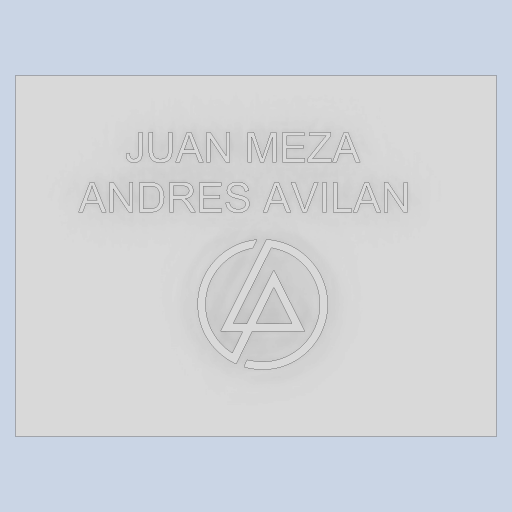
# Autodesk Inventor part: WorkObject
Saved by Autodesk Inventor 2024 (Build 280153000, 153)
## iProperties
Created: 2025-06-12
Part Number: WorkObject
Material: Genérico
Document SubType Name: Modeling
Designer: ANDRES
Density: 1 g/cm^3
Appearance: Valor por defecto
Author: ANDRES
## iProperties of the stored document WorkObject_3DPrint.ipt
Created: 2025-06-12
Part Number: WorkObject_3DPrint
Material: Genérico
Document SubType Name: Modeling
Designer: ANDRES
Density: 1 g/cm^3
Appearance: Valor por defecto
Author: ANDRES
Autodesk Inventor part; units mm, degrees
(part 1 of 2)
ref_plane "YZ Plane" through (0, 0, 0) normal (1, 0, 0) x (0, 1, 0)
ref_plane "XZ Plane" through (0, 0, 0) normal (0, 1, 0) x (-1, 0, 0)
ref_plane "XY Plane" through (0, 0, 0) normal (0, 0, 1) x (1, 0, 0)
sketch "Boceto1" plane through (0, 0, 0) normal (0, 1, 0) x (-1, 0, 0)
  line L0 (-150, 200) -> (150, 200)
  line L1 (150, 200) -> (150, -200)
  line L2 (150, -200) -> (-150, -200)
  line L3 (-150, -200) -> (-150, 200)
  line L4 (-150, 200) -> (150, -200) construction
  line L5 (150, 200) -> (-150, -200) construction
  arc A0 (56.58, 521.3157) -> (56.02, 520.4336) centre (60.6067, 518.1404) ccw
  arc A1 (56.02, 520.4336) -> (37.4805, 483.3481) centre (579507.5901, -289177.5308) ccw
  arc A2 (37.4805, 483.3481) -> (18.8463, 446.0683) centre (1035576.1763, -517151.7486) ccw
  arc A3 (18.8463, 446.0683) -> (18.6785, 445.4931) centre (20.3464, 445.3186) ccw
  line L6 (18.6785, 445.4931) -> (18.6465, 445.1876)
  line L7 (18.6465, 445.1876) -> (27.0049, 445.1038)
  arc A4 (34.672, 445.0245) -> (27.0049, 445.1038) centre (-95.3721, -11763.6751) ccw
  arc A5 (36.0643, 444.9839) -> (34.672, 445.0245) centre (34.2717, 407.4492) ccw
  arc A6 (36.6251, 444.8796) -> (36.0643, 444.9839) centre (35.9641, 442.8849) ccw
  arc A7 (36.7578, 444.638) -> (36.6251, 444.8796) centre (36.5614, 444.6873) ccw
  arc A8 (36.6714, 444.3946) -> (36.7578, 444.638) centre (35.4424, 444.9681) ccw
  arc A9 (36.1244, 443.2286) -> (36.6714, 444.3946) centre (-257.4608, 581.6629) ccw
  arc A10 (35.4755, 441.8687) -> (36.1244, 443.2286) centre (-111.5625, 512.8671) ccw
  arc A11 (34.7221, 440.3207) -> (35.4755, 441.8687) centre (-214.5818, 562.6103) ccw
  arc A12 (33.8138, 438.4691) -> (34.7221, 440.3207) centre (-15927.1151, 8269.9776) ccw
  arc A13 (32.6826, 436.164) -> (33.8138, 438.4691) centre (-38386.5339, 19290.088) ccw
  arc A14 (31.5225, 433.8001) -> (32.6826, 436.164) centre (-39365.0866, 19770.3218) ccw
  arc A15 (30.5171, 431.7521) -> (31.5225, 433.8001) centre (-22230.6082, 11360.4379) ccw
  arc A16 (29.6433, 429.9908) -> (30.5171, 431.7521) centre (-180.7952, 535.4922) ccw
  arc A17 (28.8871, 428.5078) -> (29.6433, 429.9908) centre (-78.9826, 484.4496) ccw
  arc A18 (28.2088, 427.2033) -> (28.8871, 428.5078) centre (-591.4748, 750.2321) ccw
  arc A19 (28.1348, 427.1584) -> (28.2088, 427.2033) centre (28.1348, 427.2418) ccw
  arc A20 (27.8684, 427.2434) -> (28.1348, 427.1584) centre (28.1348, 427.6184) ccw
  arc A21 (26.473, 428.2438) -> (27.8684, 427.2434) centre (142.9512, 589.2444) ccw
  arc A22 (24.9236, 429.3938) -> (26.473, 428.2438) centre (72.7691, 492.2361) ccw
  arc A23 (23.2747, 430.6746) -> (24.9236, 429.3938) centre (90.4559, 515.4667) ccw
  arc A24 (22.067, 431.7126) -> (23.2747, 430.6746) centre (35.6607, 446.3075) ccw
  arc A25 (20.3332, 433.3678) -> (22.067, 431.7126) centre (88.1482, 502.661) ccw
  arc A26 (18.6259, 435.0814) -> (20.3332, 433.3678) centre (87.4765, 501.9746) ccw
  arc A27 (17.48, 436.3457) -> (18.6259, 435.0814) centre (36.2949, 452.2481) ccw
  arc A28 (13.5474, 441.6568) -> (17.48, 436.3457) centre (56.7269, 469.5173) ccw
  arc A29 (10.3812, 447.3667) -> (13.5474, 441.6568) centre (54.6926, 468.2048) ccw
  arc A30 (8.0376, 453.3736) -> (10.3812, 447.3667) centre (53.5788, 467.6811) ccw
  arc A31 (6.5582, 459.5704) -> (8.0376, 453.3736) centre (51.4563, 467.0144) ccw
  arc A32 (5.9428, 465.5103) -> (6.5582, 459.5704) centre (54.8244, 467.5728) ccw
  arc A33 (6.0671, 471.4117) -> (5.9428, 465.5103) centre (52.6125, 467.4794) ccw
  arc A34 (6.9354, 477.2601) -> (6.0671, 471.4117) centre (52.7724, 467.4658) ccw
  arc A35 (8.5411, 483.0418) -> (6.9354, 477.2601) centre (55.5517, 466.872) ccw
  arc A36 (8.8077, 483.7953) -> (8.5411, 483.0418) centre (51.7387, 468.1835) ccw
  arc A37 (9.0978, 484.5741) -> (8.8077, 483.7953) centre (58.9745, 465.5522) ccw
  arc A38 (9.3696, 485.2705) -> (9.0978, 484.5741) centre (53.7953, 467.5275) ccw
  arc A39 (9.5686, 485.7358) -> (9.3696, 485.2705) centre (19.1573, 481.3614) ccw
  arc A40 (9.5686, 485.7358) -> (9.754, 486.1447) centre (-82.6634, 527.8125) ccw
  arc A41 (9.754, 486.1447) -> (9.9738, 486.6338) centre (-177.4212, 570.5358) ccw
  arc A42 (9.9738, 486.6338) -> (10.192, 487.1231) centre (-177.2147, 570.4436) ccw
  arc A43 (10.192, 487.1231) -> (10.3727, 487.5319) centre (-81.1266, 527.7232) ccw
  arc A44 (10.8594, 488.5609) -> (10.3727, 487.5319) centre (29.0437, 479.3306) ccw
  arc A45 (11.5431, 489.8652) -> (10.8594, 488.5609) centre (60.9878, 463.1158) ccw
  arc A46 (12.3007, 491.2233) -> (11.5431, 489.8652) centre (64.513, 461.2087) ccw
  arc A47 (13.026, 492.4363) -> (12.3007, 491.2233) centre (47.9467, 470.7319) ccw
  arc A48 (14.5448, 494.729) -> (13.026, 492.4363) centre (53.3029, 467.4029) ccw
  arc A49 (16.1634, 496.8803) -> (14.5448, 494.729) centre (50.1434, 469.6305) ccw
  arc A50 (17.9442, 498.9683) -> (16.1634, 496.8803) centre (51.5483, 468.5038) ccw
  arc A51 (19.9504, 501.071) -> (17.9442, 498.9683) centre (60.1995, 460.6608) ccw
  arc A52 (22.744, 503.6708) -> (19.9504, 501.071) centre (59.6823, 461.18) ccw
  arc A53 (25.5447, 505.9117) -> (22.744, 503.6708) centre (51.5895, 470.4893) ccw
  arc A54 (28.5205, 507.9181) -> (25.5447, 505.9117) centre (51.6227, 470.4442) ccw
  arc A55 (31.8403, 509.8131) -> (28.5205, 507.9181) centre (58.2314, 459.7244) ccw
  arc A56 (34.515, 511.0855) -> (31.8403, 509.8131) centre (48.7147, 477.7864) ccw
  arc A57 (37.6118, 512.3014) -> (34.515, 511.0855) centre (57.0679, 458.1976) ccw
  arc A58 (40.7254, 513.3196) -> (37.6118, 512.3014) centre (56.6248, 459.4299) ccw
  arc A59 (43.4452, 513.9864) -> (40.7254, 513.3196) centre (49.2545, 484.4109) ccw
  arc A60 (43.4452, 513.9864) -> (43.9181, 514.0793) centre (-966.1316, 5653.8664) ccw
  arc A61 (43.9181, 514.0793) -> (44.3678, 514.1677) centre (-805.8341, 4838.1588) ccw
  arc A62 (44.3678, 514.1677) -> (44.7484, 514.2425) centre (-769.0566, 4651.0806) ccw
  arc A63 (44.7484, 514.2425) -> (44.9368, 514.2797) centre (-13.5465, 810.5736) ccw
  arc A64 (44.9368, 514.2797) -> (45.1645, 514.4286) centre (44.8666, 514.6354) ccw
  arc A65 (45.1645, 514.4286) -> (45.5138, 514.9782) centre (38.5801, 518.9988) ccw
  arc A66 (45.5138, 514.9782) -> (46.021, 515.9115) centre (28.9096, 524.6064) ccw
  arc A67 (46.021, 515.9115) -> (46.9084, 517.6797) centre (-131.1326, 605.9294) ccw
  arc A68 (46.9084, 517.6797) -> (47.5391, 518.9693) centre (-74.896, 578.0546) ccw
  arc A69 (47.5391, 518.9693) -> (48.0629, 520.0783) centre (-17.9294, 550.5634) ccw
  arc A70 (48.0629, 520.0783) -> (48.5097, 521.0508) centre (-192.1871, 631.0618) ccw
  arc A71 (48.5097, 521.0508) -> (48.5155, 521.1586) centre (48.3757, 521.112) ccw
  arc A72 (48.5155, 521.1586) -> (48.2718, 521.3168) centre (48.2945, 521.085) ccw
  arc A73 (48.2718, 521.3168) -> (46.7225, 521.1428) centre (53.5837, 467.0473) ccw
  arc A74 (46.7225, 521.1428) -> (44.7418, 520.841) centre (51.7639, 481.3956) ccw
  arc A75 (44.7418, 520.841) -> (42.2018, 520.3578) centre (63.9176, 413.1243) ccw
  arc A76 (42.2018, 520.3578) -> (32.5036, 517.3294) centre (52.0213, 471.8684) ccw
  arc A77 (32.5036, 517.3294) -> (23.3662, 512.3255) centre (54.057, 467.1269) ccw
  arc A78 (23.3662, 512.3255) -> (15.258, 505.6197) centre (54.6829, 466.2051) ccw
  arc A79 (15.258, 505.6197) -> (8.6097, 497.548) centre (53.7288, 467.1589) ccw
  arc A80 (8.6097, 497.548) -> (7.5165, 495.8912) centre (95.1179, 439.2823) ccw
  arc A81 (7.5165, 495.8912) -> (6.7388, 494.6269) centre (35.5048, 477.8049) ccw
  arc A82 (6.7388, 494.6269) -> (6.0239, 493.3384) centre (34.9485, 478.1302) ccw
  arc A83 (6.0239, 493.3384) -> (5.1357, 491.6074) centre (92.2684, 447.9919) ccw
  arc A84 (5.1357, 491.6074) -> (3.5381, 488.146) centre (58.912, 464.6889) ccw
  arc A85 (3.5381, 488.146) -> (2.2189, 484.701) centre (52.1007, 467.5742) ccw
  arc A86 (2.2189, 484.701) -> (1.1783, 481.2726) centre (49.2418, 468.5559) ccw
  arc A87 (1.1783, 481.2726) -> (0.4159, 477.8611) centre (44.7392, 469.7472) ccw
  arc A88 (0.3239, 477.3608) -> (0.4159, 477.8611) centre (-293.8796, 531.7347) ccw
  arc A89 (0.2252, 476.8288) -> (0.3239, 477.3608) centre (-376.5295, 547.01) ccw
  arc A90 (0.134, 476.3415) -> (0.2252, 476.8288) centre (-342.0128, 540.5806) ccw
  arc A91 (0.0685, 475.996) -> (0.134, 476.3415) centre (-89.414, 493.1544) ccw
  arc A92 (0.0685, 475.996) -> (-0.1998, 474.1813) centre (21.1882, 471.9462) ccw
  arc A93 (-0.1998, 474.1813) -> (-0.3729, 471.9952) centre (43.2094, 469.645) ccw
  arc A94 (-0.3729, 471.9952) -> (-0.4555, 469.4334) centre (58.7799, 468.8053) ccw
  arc A95 (-0.4555, 469.4334) -> (-0.4456, 466.4633) centre (106.0144, 468.3044) ccw
  arc A96 (-0.4456, 466.4633) -> (-0.2833, 462.3774) centre (90.7872, 468.0411) ccw
  arc A97 (-0.2833, 462.3774) -> (0.0608, 459.1163) centre (37.7893, 464.7451) ccw
  arc A98 (0.0608, 459.1163) -> (0.6935, 455.817) centre (40.2126, 465.1067) ccw
  arc A99 (0.6935, 455.817) -> (1.774, 451.5865) centre (111.5521, 481.8763) ccw
  arc A100 (1.774, 451.5865) -> (2.11, 450.5047) centre (18.8675, 456.303) ccw
  arc A101 (2.11, 450.5047) -> (2.6756, 448.923) centre (79.2137, 477.1836) ccw
  arc A102 (2.6756, 448.923) -> (3.3191, 447.2351) centre (83.2059, 478.6577) ccw
  arc A103 (3.3191, 447.2351) -> (3.9298, 445.7479) centre (53.5125, 466.9782) ccw
  arc A104 (3.9298, 445.7479) -> (7.8799, 438.3689) centre (48.2347, 464.7183) ccw
  arc A105 (7.8799, 438.3689) -> (13.2128, 431.4158) centre (56.3004, 469.9847) ccw
  arc A106 (13.2128, 431.4158) -> (19.5475, 425.3345) centre (56.4761, 470.1419) ccw
  arc A107 (19.5475, 425.3345) -> (26.4828, 420.5527) centre (50.8578, 463.3249) ccw
  arc A108 (26.4828, 420.5527) -> (28.232, 419.5861) centre (64.0229, 486.4265) ccw
  arc A109 (28.232, 419.5861) -> (29.7435, 418.8181) centre (46.8541, 454.3634) ccw
  arc A110 (29.7435, 418.8181) -> (31.007, 418.2282) centre (55.3367, 471.9851) ccw
  arc A111 (31.007, 418.2282) -> (31.3314, 418.2187) centre (31.1806, 418.6117) ccw
  arc A112 (31.3314, 418.2187) -> (31.4578, 418.3289) centre (31.2441, 418.4462) ccw
  arc A113 (31.4578, 418.3289) -> (32.0217, 419.3658) centre (-106.2153, 493.8829) ccw
  arc A114 (32.0217, 419.3658) -> (32.6587, 420.5802) centre (-21.1358, 448.0204) ccw
  arc A115 (32.6587, 420.5802) -> (33.3727, 422.0054) centre (-65.2475, 470.5215) ccw
  arc A116 (34.237, 423.7622) -> (33.3727, 422.0054) centre (48832.2866, -23584.636) ccw
  arc A117 (35.348, 426.0203) -> (34.237, 423.7622) centre (141170.8048, -69014.9686) ccw
  arc A118 (36.5085, 428.379) -> (35.348, 426.0203) centre (147450.9926, -72105.2267) ccw
  arc A119 (37.5394, 430.4741) -> (36.5085, 428.379) centre (87335.0324, -42525.9942) ccw
  arc A120 (37.5394, 430.4741) -> (38.5161, 432.4611) centre (-2251.0652, 1556.6292) ccw
  arc A121 (38.5161, 432.4611) -> (39.5111, 434.4897) centre (-2447.0255, 1652.844) ccw
  arc A122 (39.5111, 434.4897) -> (40.3917, 436.2887) centre (-2175.5651, 1519.8339) ccw
  arc A123 (40.3917, 436.2887) -> (40.9579, 437.4509) centre (-370.305, 637.1084) ccw
  arc A124 (41.4639, 438.4928) -> (40.9579, 437.4509) centre (3561.0942, -1271.4826) ccw
  arc A125 (42.1073, 439.8168) -> (41.4639, 438.4928) centre (8987.4877, -3907.8382) ccw
  arc A126 (42.7752, 441.1908) -> (42.1073, 439.8168) centre (9584.0231, -4197.7703) ccw
  arc A127 (43.3637, 442.4008) -> (42.7752, 441.1908) centre (5750.8793, -2334.1005) ccw
  line L8 (43.3637, 442.4008) -> (44.6963, 445.1402)
  line L9 (44.6963, 445.1402) -> (66.4506, 445.1052)
  arc A128 (66.4506, 445.1052) -> (74.7976, 445.0973) centre (76.5381, 6711.6022) ccw
  arc A129 (74.7976, 445.0973) -> (81.8373, 445.1032) centre (75.68, 3627.6056) ccw
  arc A130 (81.8373, 445.1032) -> (88.2058, 445.1157) centre (-99.4327, 94099.4853) ccw
  arc A131 (88.2058, 445.1157) -> (88.2822, 445.1474) centre (88.2056, 445.2241) ccw
  arc A132 (88.2822, 445.1474) -> (88.3144, 445.327) centre (88.1693, 445.2603) ccw
  arc A133 (88.3144, 445.327) -> (87.5678, 446.9366) centre (-128.8707, 345.5653) ccw
  arc A134 (87.5678, 446.9366) -> (86.5747, 448.9963) centre (-4.4011, 403.8619) ccw
  arc A135 (86.5747, 448.9963) -> (85.1252, 451.888) centre (-265.2635, 274.4445) ccw
  arc A136 (84.0923, 453.9304) -> (85.1252, 451.888) centre (1934.5298, 1388.4612) ccw
  arc A137 (82.4268, 457.2294) -> (84.0923, 453.9304) centre (11699.7284, 6320.2032) ccw
  arc A138 (80.528, 460.9933) -> (82.4268, 457.2294) centre (13150.3703, 7052.2983) ccw
  arc A139 (78.6409, 464.7364) -> (80.528, 460.9933) centre (12725.2516, 6837.9109) ccw
  arc A140 (78.6409, 464.7364) -> (72.7933, 476.3341) centre (-27537.7918, -13452.4177) ccw
  arc A141 (72.7933, 476.3341) -> (68.3879, 485.0562) centre (-8939.9079, -4070.3134) ccw
  arc A142 (68.3879, 485.0562) -> (65.0873, 491.5735) centre (-5364.3361, -2262.194) ccw
  arc A143 (65.0873, 491.5735) -> (62.9668, 495.7323) centre (-903.1215, 0.5055) ccw
  arc A144 (62.9668, 495.7323) -> (62.8365, 495.9737) centre (57.2457, 492.7996) ccw
  arc A145 (62.8365, 495.9737) -> (62.7681, 496.0314) centre (62.7238, 495.9097) ccw
  arc A146 (62.7681, 496.0314) -> (62.6993, 496.0139) centre (62.7465, 495.9722) ccw
  arc A147 (62.6993, 496.0139) -> (62.5868, 495.8704) centre (63.8582, 494.9901) ccw
  arc A148 (62.5868, 495.8704) -> (62.1739, 495.177) centre (67.4296, 492.5171) ccw
  arc A149 (62.1739, 495.177) -> (59.2866, 489.4641) centre (5235.4295, -2122.9744) ccw
  arc A150 (59.2866, 489.4641) -> (55.3949, 481.7242) centre (2613.4519, -799.6406) ccw
  arc A151 (55.3949, 481.7242) -> (49.3635, 469.6704) centre (14068.3573, -6537.5657) ccw
  line L10 (49.3635, 469.6704) -> (40.2528, 451.4433)
  line L11 (40.2528, 451.4433) -> (34.7406, 451.4934)
  arc A152 (32.1516, 451.525) -> (34.7406, 451.4934) centre (38.4834, 863.5141) ccw
  arc A153 (30.4729, 451.569) -> (32.1516, 451.525) centre (33.3438, 529.1012) ccw
  arc A154 (29.2549, 451.6208) -> (30.4729, 451.569) centre (34.5532, 561.7611) ccw
  arc A155 (29.0684, 451.7034) -> (29.2549, 451.6208) centre (29.2685, 451.9035) ccw
  arc A156 (29.0267, 451.9573) -> (29.0684, 451.7034) centre (29.2244, 451.8594) ccw
  arc A157 (32.2865, 458.5362) -> (29.0267, 451.9573) centre (7472.7976, -3232.3522) ccw
  arc A158 (36.6719, 467.3028) -> (32.2865, 458.5362) centre (1339.8045, -190.0614) ccw
  arc A159 (43.8601, 481.5221) -> (36.6719, 467.3028) centre (8404.6001, -3753.8908) ccw
  arc A160 (43.8601, 481.5221) -> (45.1995, 484.1688) centre (-3214.8736, 2132.3428) ccw
  arc A161 (45.1995, 484.1688) -> (47.0258, 487.7827) centre (-10971.9126, 6054.0265) ccw
  arc A162 (47.0258, 487.7827) -> (48.9906, 491.6738) centre (-11961.6818, 6554.0163) ccw
  arc A163 (48.9906, 491.6738) -> (50.8041, 495.2685) centre (-8675.0157, 4895.0902) ccw
  arc A164 (56.379, 506.3138) -> (50.8041, 495.2685) centre (13791.4775, -6433.2201) ccw
  arc A165 (58.8082, 511.0773) -> (56.379, 506.3138) centre (694.0923, 184.1148) ccw
  arc A166 (60.3319, 514.0208) -> (58.8082, 511.0773) centre (681.0708, 190.8171) ccw
  arc A167 (60.6355, 514.3709) -> (60.3319, 514.0208) centre (61.2173, 513.5597) ccw
  arc A168 (61.3554, 514.5147) -> (60.6355, 514.3709) centre (61.1543, 513.6476) ccw
  arc A169 (64.443, 513.7578) -> (61.3554, 514.5147) centre (32.8545, 391.5787) ccw
  arc A170 (67.7144, 512.8196) -> (64.443, 513.7578) centre (48.2469, 451.1141) ccw
  arc A171 (70.6723, 511.776) -> (67.7144, 512.8196) centre (53.6569, 468.2619) ccw
  arc A172 (77.6775, 508.3629) -> (70.6723, 511.776) centre (53.0524, 466.7159) ccw
  arc A173 (84.0145, 503.8812) -> (77.6775, 508.3629) centre (53.4366, 467.3656) ccw
  arc A174 (89.5104, 498.4539) -> (84.0145, 503.8812) centre (53.7392, 467.727) ccw
  arc A175 (94.0148, 492.2291) -> (89.5104, 498.4539) centre (54.477, 468.3608) ccw
  arc A176 (94.8641, 490.7345) -> (94.0148, 492.2291) centre (66.1123, 475.3848) ccw
  arc A177 (95.8933, 488.749) -> (94.8641, 490.7345) centre (13.876, 447.4976) ccw
  arc A178 (96.8674, 486.7522) -> (95.8933, 488.749) centre (14.1139, 447.6172) ccw
  arc A179 (97.535, 485.2303) -> (96.8674, 486.7522) centre (70.3919, 474.2316) ccw
  arc A180 (97.535, 485.2303) -> (97.7339, 484.7424) centre (210.1585, 530.8667) ccw
  arc A181 (97.7339, 484.7424) -> (97.9223, 484.2865) centre (184.1006, 520.1758) ccw
  arc A182 (97.9223, 484.2865) -> (98.0827, 483.9038) centre (184.4264, 520.3114) ccw
  arc A183 (98.0827, 483.9038) -> (98.1587, 483.7326) centre (102.7285, 485.8628) ccw
  arc A184 (98.4052, 483.1091) -> (98.1587, 483.7326) centre (93.0699, 481.3605) ccw
  arc A185 (98.8941, 481.5865) -> (98.4052, 483.1091) centre (-27.9794, 441.6867) ccw
  arc A186 (99.3675, 480.0376) -> (98.8941, 481.5865) centre (3.2804, 451.5173) ccw
  arc A187 (99.6576, 478.9663) -> (99.3675, 480.0376) centre (77.229, 473.4665) ccw
  arc A188 (100.2025, 476.3449) -> (99.6576, 478.9663) centre (63.0398, 469.9871) ccw
  arc A189 (100.5634, 473.6777) -> (100.2025, 476.3449) centre (62.2524, 469.8524) ccw
  arc A190 (100.7676, 470.7081) -> (100.5634, 473.6777) centre (52.5837, 468.887) ccw
  arc A191 (100.8371, 467.1541) -> (100.7676, 470.7081) centre (3.3349, 467.0256) ccw
  arc A192 (100.8137, 464.5948) -> (100.8371, 467.1541) centre (-21.5806, 466.9929) ccw
  arc A193 (100.7319, 462.5658) -> (100.8137, 464.5948) centre (51.7656, 465.5558) ccw
  arc A194 (100.586, 460.8861) -> (100.7319, 462.5658) centre (67.8884, 464.5713) ccw
  arc A195 (100.3646, 459.4175) -> (100.586, 460.8861) centre (80.8443, 463.1111) ccw
  arc A196 (99.9562, 457.3179) -> (100.3646, 459.4175) centre (-104.2331, 498.1316) ccw
  arc A197 (99.6758, 456.0551) -> (99.9562, 457.3179) centre (70.0463, 463.2964) ccw
  arc A198 (99.3662, 454.914) -> (99.6758, 456.0551) centre (76.9674, 461.6049) ccw
  arc A199 (98.879, 453.3387) -> (99.3662, 454.914) centre (17.2283, 479.4498) ccw
  arc A200 (98.5246, 452.2892) -> (98.879, 453.3387) centre (66.245, 463.7747) ccw
  arc A201 (98.0921, 451.1156) -> (98.5246, 452.2892) centre (46.1396, 470.9286) ccw
  arc A202 (97.5796, 449.8114) -> (98.0921, 451.1156) centre (33.0044, 475.938) ccw
  arc A203 (96.9823, 448.3651) -> (97.5796, 449.8114) centre (-2.7096, 490.3877) ccw
  arc A204 (96.2285, 446.7313) -> (96.9823, 448.3651) centre (72.1166, 458.8467) ccw
  arc A205 (95.1222, 444.6065) -> (96.2285, 446.7313) centre (22.0442, 484.0062) ccw
  arc A206 (93.9535, 442.5119) -> (95.1222, 444.6065) centre (22.0143, 484.0224) ccw
  arc A207 (92.9973, 440.9739) -> (93.9535, 442.5119) centre (70.0923, 456.2804) ccw
  arc A208 (92.5266, 440.3022) -> (92.9973, 440.9739) centre (77.6243, 451.2471) ccw
  arc A209 (91.6073, 439.0607) -> (92.5266, 440.3022) centre (-67.8348, 558.0782) ccw
  arc A210 (90.6521, 437.7873) -> (91.6073, 439.0607) centre (-175.9394, 638.7745) ccw
  arc A211 (90.3553, 437.4344) -> (90.6521, 437.7873) centre (87.1955, 440.3933) ccw
  arc A212 (90.3553, 437.4344) -> (90.2674, 437.3364) centre (92.544, 435.3848) ccw
  arc A213 (90.2674, 437.3364) -> (90.0716, 437.1069) centre (137.5468, 396.8087) ccw
  arc A214 (90.0716, 437.1069) -> (89.84, 436.8324) centre (136.4114, 397.7725) ccw
  arc A215 (89.84, 436.8324) -> (89.593, 436.5364) centre (151.6855, 384.9621) ccw
  arc A216 (88.4794, 435.2751) -> (89.593, 436.5364) centre (68.1163, 454.3751) ccw
  arc A217 (87.0215, 433.769) -> (88.4794, 435.2751) centre (39.9292, 480.8137) ccw
  arc A218 (85.488, 432.2814) -> (87.0215, 433.769) centre (38.8643, 481.8776) ccw
  arc A219 (84.1317, 431.0696) -> (85.488, 432.2814) centre (60.8901, 458.4476) ccw
  arc A220 (77.3541, 426.2853) -> (84.1317, 431.0696) centre (53.9922, 466.5732) ccw
  arc A221 (69.7937, 422.7449) -> (77.3541, 426.2853) centre (53.4031, 467.5892) ccw
  arc A222 (61.7147, 420.569) -> (69.7937, 422.7449) centre (53.3285, 467.7934) ccw
  arc A223 (53.3974, 419.8363) -> (61.7147, 420.569) centre (53.3974, 467.4061) ccw
  arc A224 (50.8363, 419.9016) -> (53.3974, 419.8363) centre (53.3974, 470.0384) ccw
  arc A225 (48.39, 420.0979) -> (50.8363, 419.9016) centre (52.9934, 462.1277) ccw
  arc A226 (45.7794, 420.4541) -> (48.39, 420.0979) centre (53.8035, 469.525) ccw
  arc A227 (42.7069, 421.0071) -> (45.7794, 420.4541) centre (61.5143, 516.6798) ccw
  arc A228 (42.7069, 421.0071) -> (42.0093, 421.1407) centre (28.5654, 349.0694) ccw
  arc A229 (42.0093, 421.1407) -> (41.3817, 421.2535) centre (33.2649, 374.2628) ccw
  arc A230 (41.3817, 421.2535) -> (40.8534, 421.3424) centre (30.624, 358.9736) ccw
  arc A231 (40.8534, 421.3424) -> (40.6874, 421.3559) centre (40.6874, 420.3302) ccw
  arc A232 (40.6874, 421.3559) -> (40.4362, 421.2109) centre (40.6874, 421.0659) ccw
  arc A233 (40.4362, 421.2109) -> (39.8616, 420.1725) centre (68.7677, 404.8561) ccw
  arc A234 (39.8616, 420.1725) -> (39.2205, 418.8703) centre (61.4065, 408.7566) ccw
  arc A235 (39.2205, 418.8703) -> (38.5504, 417.3228) centre (79.4988, 400.5091) ccw
  arc A236 (38.5504, 417.3228) -> (38.2002, 416.4192) centre (61.0077, 408.1017) ccw
  arc A237 (38.2002, 416.4192) -> (38.0851, 415.9285) centre (40.1903, 415.6934) ccw
  arc A238 (38.0851, 415.9285) -> (38.1358, 415.625) centre (38.6452, 415.866) ccw
  arc A239 (38.1358, 415.625) -> (38.3372, 415.4134) centre (38.5571, 415.8243) ccw
  arc A240 (38.3372, 415.4134) -> (39.0723, 415.1427) centre (39.6749, 417.913) ccw
  arc A241 (39.0723, 415.1427) -> (41.3208, 414.6744) centre (66.6082, 541.716) ccw
  arc A242 (41.3208, 414.6744) -> (43.9738, 414.1824) centre (61.3616, 515.357) ccw
  arc A243 (43.9738, 414.1824) -> (46.83, 413.7229) centre (66.9449, 547.8432) ccw
  arc A244 (46.83, 413.7229) -> (48.1113, 413.5569) centre (51.6045, 445.5574) ccw
  arc A245 (48.1113, 413.5569) -> (49.2358, 413.4683) centre (50.1464, 432.2003) ccw
  arc A246 (49.2358, 413.4683) -> (50.6187, 413.4303) centre (50.8278, 446.2164) ccw
  arc A247 (50.6187, 413.4303) -> (52.9088, 413.4274) centre (52.0516, 638.1193) ccw
  arc A248 (52.9088, 413.4274) -> (56.1284, 413.4866) centre (52.4881, 523.7435) ccw
  arc A249 (56.1284, 413.4866) -> (58.8592, 413.6417) centre (54.2255, 471.1227) ccw
  arc A250 (58.8592, 413.6417) -> (61.317, 413.9062) centre (55.1474, 459.6866) ccw
  arc A251 (61.317, 413.9062) -> (63.6999, 414.2973) centre (55.6993, 455.592) ccw
  arc A252 (63.6999, 414.2973) -> (75.4933, 418.0271) centre (53.443, 467.2377) ccw
  arc A253 (75.4933, 418.0271) -> (86.1346, 424.3478) centre (53.3874, 467.3618) ccw
  arc A254 (86.1346, 424.3478) -> (95.0675, 432.9292) centre (53.332, 467.4344) ccw
  arc A255 (95.0675, 432.9292) -> (101.825, 443.3225) centre (53.199, 467.5444) ccw
  arc A256 (101.825, 443.3225) -> (103.4148, 446.8684) centre (59.0379, 464.6358) ccw
  arc A257 (103.4148, 446.8684) -> (104.8322, 450.7796) centre (45.1722, 470.1873) ccw
  arc A258 (104.8322, 450.7796) -> (105.9707, 454.7237) centre (46.5261, 469.7469) ccw
  arc A259 (105.9707, 454.7237) -> (106.7189, 458.3664) centre (65.8776, 464.8563) ccw
  arc A260 (106.8302, 459.0637) -> (106.7189, 458.3664) centre (530.9092, 390.9607) ccw
  arc A261 (106.936, 459.7183) -> (106.8302, 459.0637) centre (436.8265, 406.07) ccw
  arc A262 (107.0261, 460.2694) -> (106.936, 459.7183) centre (434.2095, 406.4961) ccw
  arc A263 (107.0695, 460.5227) -> (107.0261, 460.2694) centre (125.8059, 457.1829) ccw
  arc A264 (107.0695, 460.5227) -> (107.1855, 461.4318) centre (97.9498, 462.1483) ccw
  arc A265 (107.1855, 461.4318) -> (107.359, 463.7953) centre (-177.4827, 483.5164) ccw
  arc A266 (107.359, 463.7953) -> (107.5086, 466.1379) centre (-110.5236, 478.8804) ccw
  arc A267 (107.5086, 466.1379) -> (107.5478, 467.4304) centre (84.495, 467.4829) ccw
  arc A268 (107.5478, 467.4304) -> (107.4362, 470.5895) centre (65.482, 467.5262) ccw
  arc A269 (107.4362, 470.5895) -> (107.0843, 474.0912) centre (43.0814, 465.8906) ccw
  arc A270 (107.0843, 474.0912) -> (106.5383, 477.5951) centre (42.267, 465.7863) ccw
  arc A271 (106.5383, 477.5951) -> (105.8396, 480.7623) centre (61.5163, 469.323) ccw
  arc A272 (105.8396, 480.7623) -> (104.0299, 486.4934) centre (51.2083, 466.6626) ccw
  arc A273 (104.0299, 486.4934) -> (101.6412, 491.9203) centre (53.9781, 467.7024) ccw
  arc A274 (101.6412, 491.9203) -> (98.6738, 497.0345) centre (54.2536, 467.8424) ccw
  arc A275 (98.6738, 497.0345) -> (95.1345, 501.8308) centre (52.7962, 466.8847) ccw
  arc A276 (95.1345, 501.8308) -> (89.3045, 507.8849) centre (52.7322, 466.8319) ccw
  arc A277 (89.3045, 507.8849) -> (82.6069, 512.9951) centre (52.3896, 466.4472) ccw
  arc A278 (82.6069, 512.9951) -> (75.3088, 516.9704) centre (53.2036, 467.7009) ccw
  arc A279 (75.3088, 516.9704) -> (67.6913, 519.646) centre (55.6027, 473.0482) ccw
  arc A280 (67.6913, 519.646) -> (64.3011, 520.4219) centre (52.5343, 461.2204) ccw
  arc A281 (64.3011, 520.4219) -> (60.6344, 521.0615) centre (48.8756, 442.8121) ccw
  arc A282 (60.6344, 521.0615) -> (57.1587, 521.551) centre (32.4142, 333.2702) ccw
  arc A283 (57.1587, 521.551) -> (56.58, 521.3157) centre (57.0763, 520.9243) ccw
  arc A284 (68.4755, 470.5774) -> (64.224, 478.9413) centre (-1012.5795, -73.6764) ccw
  arc A285 (73.0645, 461.3946) -> (68.4755, 470.5774) centre (-1479.3174, -308.657) ccw
  arc A286 (77.7625, 451.9205) -> (73.0645, 461.3946) centre (-34251.2399, -16565.065) ccw
  arc A287 (77.7289, 451.7161) -> (77.7625, 451.9205) centre (77.6034, 451.8416) ccw
  arc A288 (77.4045, 451.5805) -> (77.7289, 451.7161) centre (77.4016, 452.0434) ccw
  arc A289 (66.8078, 451.5178) -> (77.4045, 451.5805) centre (-66.657, 23895.5299) ccw
  arc A290 (57.4227, 451.4925) -> (66.8078, 451.5178) centre (57.8926, 2017.7716) ccw
  arc A291 (52.0108, 451.5697) -> (57.4227, 451.4925) centre (57.4809, 645.3585) ccw
  arc A292 (49.5477, 451.6448) -> (52.0108, 451.5697) centre (67.3122, 993.6652) ccw
  arc A293 (48.6496, 451.7019) -> (49.5477, 451.6448) centre (50.0268, 466.2638) ccw
  arc A294 (48.215, 451.7832) -> (48.6496, 451.7019) centre (48.8794, 454.1318) ccw
  arc A295 (48.1175, 451.9379) -> (48.215, 451.7832) centre (48.2522, 451.9148) ccw
  arc A296 (48.2233, 452.2724) -> (48.1175, 451.9379) centre (49.3886, 451.7198) ccw
  arc A297 (49.0583, 454.0227) -> (48.2233, 452.2724) centre (428.4792, 271.9399) ccw
  arc A298 (50.3286, 456.6449) -> (49.0583, 454.0227) centre (407.7243, 281.9001) ccw
  arc A299 (52.7014, 461.4898) -> (50.3286, 456.6449) centre (3677.8948, -1317.019) ccw
  arc A300 (52.7014, 461.4898) -> (54.6312, 465.4264) centre (-6463.9677, 3658.5504) ccw
  arc A301 (54.6312, 465.4264) -> (56.2666, 468.7691) centre (-3341.5996, 2129.0665) ccw
  arc A302 (56.2666, 468.7691) -> (57.6082, 471.5188) centre (-2338.2325, 1638.7912) ccw
  arc A303 (57.6082, 471.5188) -> (58.6082, 473.5783) centre (-709.2156, 845.1204) ccw
  arc A304 (61.0981, 478.7108) -> (58.6082, 473.5783) centre (2626.1322, -768.8168) ccw
  arc A305 (62.0456, 480.5954) -> (61.0981, 478.7108) centre (133.1066, 443.6888) ccw
  arc A306 (62.5991, 481.6116) -> (62.0456, 480.5954) centre (88.0317, 467.0991) ccw
  arc A307 (62.7926, 481.6349) -> (62.5991, 481.6116) centre (62.7045, 481.5514) ccw
  arc A308 (62.8613, 481.5396) -> (62.7926, 481.6349) centre (62.4729, 481.3318) ccw
  arc A309 (63.2571, 480.7971) -> (62.8613, 481.5396) centre (-215.2181, 332.8132) ccw
  arc A310 (63.7086, 479.9386) -> (63.2571, 480.7971) centre (-35.3803, 428.3805) ccw
  arc A311 (64.224, 478.9413) -> (63.7086, 479.9386) centre (-113.4969, 387.7347) ccw
  line L12 (-53.5181, 588.2642) -> (-54.5646, 588.3838)
  line L13 (-54.5646, 588.3838) -> (-56.1493, 589.3106)
  line L14 (-56.1493, 589.3106) -> (-56.239, 589.4302)
  line L15 (-56.239, 589.4302) -> (-56.8968, 590.8953)
  line L16 (-56.8968, 590.8953) -> (-57.1958, 593.1976)
  line L17 (-57.1958, 593.1976) -> (-60.1558, 592.779)
  line L18 (-60.1558, 592.779) -> (-60.1558, 592.5697)
  line L19 (-60.1558, 592.5697) -> (-59.9764, 590.4169)
  line L20 (-59.9764, 590.4169) -> (-59.4083, 588.623)
  line L21 (-59.4083, 588.623) -> (-58.4814, 587.2177)
  line L22 (-58.4814, 587.2177) -> (-57.3154, 586.2609)
  line L23 (-57.3154, 586.2609) -> (-55.6111, 585.5732)
  line L24 (-55.6111, 585.5732) -> (-53.5181, 585.334)
  line L25 (-53.5181, 585.334) -> (-53.4583, 585.334)
  line L26 (-53.4583, 585.334) -> (-51.4252, 585.5732)
  line L27 (-51.4252, 585.5732) -> (-49.691, 586.231)
  line L28 (-49.691, 586.231) -> (-48.3754, 587.2177)
  line L29 (-48.3754, 587.2177) -> (-47.2991, 588.8322)
  line L30 (-47.2991, 588.8322) -> (-47.0599, 589.5797)
  line L31 (-47.0599, 589.5797) -> (-46.7011, 591.3737)
  line L32 (-46.7011, 591.3737) -> (-46.5815, 593.646)
  line L33 (-46.5815, 593.646) -> (-46.5815, 610.4794)
  line L34 (-46.5815, 610.4794) -> (-49.8405, 610.4794)
  line L35 (-49.8405, 610.4794) -> (-49.8405, 593.4666)
  line L36 (-49.8405, 593.4666) -> (-49.8704, 592.0614)
  line L37 (-49.8704, 592.0614) -> (-50.1694, 590.3571)
  line L38 (-50.1694, 590.3571) -> (-50.1993, 590.2973)
  line L39 (-50.1993, 590.2973) -> (-51.3953, 588.8322)
  line L40 (-51.3953, 588.8322) -> (-51.6345, 588.7126)
  line L41 (-51.6345, 588.7126) -> (-53.5181, 588.2642)
  line L42 (-38.6582, 587.6961) -> (-37.0735, 586.53)
  line L43 (-37.0735, 586.53) -> (-35.4589, 585.8722)
  line L44 (-35.4589, 585.8722) -> (-33.5753, 585.4835)
  line L45 (-33.5753, 585.4835) -> (-31.3926, 585.334)
  line L46 (-31.3926, 585.334) -> (-31.1833, 585.334)
  line L47 (-31.1833, 585.334) -> (-29.0605, 585.5134)
  line L48 (-29.0605, 585.5134) -> (-27.1768, 585.9918)
  line L49 (-27.1768, 585.9918) -> (-25.622, 586.7393)
  line L50 (-25.622, 586.7393) -> (-24.8446, 587.2476)
  line L51 (-24.8446, 587.2476) -> (-23.4992, 588.623)
  line L52 (-23.4992, 588.623) -> (-22.5723, 590.2973)
  line L53 (-22.5723, 590.2973) -> (-22.5424, 590.3571)
  line L54 (-22.5424, 590.3571) -> (-22.0939, 592.0016)
  line L55 (-22.0939, 592.0016) -> (-21.8248, 593.945)
  line L56 (-21.8248, 593.945) -> (-21.7351, 596.2174)
  line L57 (-21.7351, 596.2174) -> (-21.7351, 610.4794)
  line L58 (-21.7351, 610.4794) -> (-25.024, 610.4794)
  line L59 (-25.024, 610.4794) -> (-25.024, 596.2174)
  line L60 (-25.024, 596.2174) -> (-25.024, 595.141)
  line L61 (-25.024, 595.141) -> (-25.2632, 592.8687)
  line L62 (-25.2632, 592.8687) -> (-25.7715, 591.1345)
  line L63 (-25.7715, 591.1345) -> (-26.5489, 589.9385)
  line L64 (-26.5489, 589.9385) -> (-27.6851, 589.0714)
  line L65 (-27.6851, 589.0714) -> (-29.4491, 588.5034)
  line L66 (-29.4491, 588.5034) -> (-31.6916, 588.2941)
  line L67 (-31.6916, 588.2941) -> (-33.5155, 588.4735)
  line L68 (-33.5155, 588.4735) -> (-35.2496, 589.1312)
  line L69 (-35.2496, 589.1312) -> (-36.2662, 589.8787)
  line L70 (-36.2662, 589.8787) -> (-37.3127, 591.4933)
  line L71 (-37.3127, 591.4933) -> (-37.4921, 592.0913)
  line L72 (-37.4921, 592.0913) -> (-37.7911, 593.8852)
  line L73 (-37.7911, 593.8852) -> (-37.9107, 596.2174)
  line L74 (-37.9107, 596.2174) -> (-37.9107, 610.4794)
  line L75 (-37.9107, 610.4794) -> (-41.1697, 610.4794)
  line L76 (-41.1697, 610.4794) -> (-41.1697, 596.2174)
  line L77 (-41.1697, 596.2174) -> (-41.1697, 595.7091)
  line L78 (-41.1697, 595.7091) -> (-41.0501, 593.4965)
  line L79 (-41.0501, 593.4965) -> (-40.7212, 591.583)
  line L80 (-40.7212, 591.583) -> (-40.2428, 590.0282)
  line L81 (-40.2428, 590.0282) -> (-39.8242, 589.191)
  line L82 (-39.8242, 589.191) -> (-38.6582, 587.6961)
  line L83 (-11.8683, 595.9184) -> (-9.1774, 603.1839)
  line L84 (-9.1774, 603.1839) -> (-8.8485, 604.0809)
  line L85 (-8.8485, 604.0809) -> (-8.2804, 605.9945)
  line L86 (-8.2804, 605.9945) -> (-7.8319, 607.908)
  line L87 (-6.008, 610.4794) -> (-9.5362, 610.4794)
  line L88 (-9.5362, 610.4794) -> (-19.0143, 585.7526)
  line L89 (-19.0143, 585.7526) -> (-15.5459, 585.7526)
  line L90 (-15.5459, 585.7526) -> (-12.8251, 593.2574)
  line L91 (-12.8251, 593.2574) -> (-2.4799, 593.2574)
  line L92 (-2.4799, 593.2574) -> (0.3904, 585.7526)
  line L93 (0.3904, 585.7526) -> (4.1279, 585.7526)
  line L94 (4.1279, 585.7526) -> (-6.008, 610.4794)
  line L95 (-7.8319, 607.908) -> (-7.4731, 606.7121)
  line L96 (-7.4731, 606.7121) -> (-6.8751, 604.8882)
  line L97 (-6.8751, 604.8882) -> (-6.0977, 602.7654)
  line L98 (-6.0977, 602.7654) -> (-3.4965, 595.9184)
  line L99 (-3.4965, 595.9184) -> (-11.8683, 595.9184)
  line L100 (22.815, 585.7526) -> (26.1637, 585.7526)
  line L101 (26.1637, 585.7526) -> (26.1637, 610.4794)
  line L102 (26.1637, 610.4794) -> (23.0243, 610.4794)
  line L103 (23.0243, 610.4794) -> (23.0243, 591.0747)
  line L104 (10.0479, 610.4794) -> (6.6992, 610.4794)
  line L105 (6.6992, 610.4794) -> (6.6992, 585.7526)
  line L106 (6.6992, 585.7526) -> (9.8386, 585.7526)
  line L107 (9.8386, 585.7526) -> (9.8386, 605.1872)
  line L108 (23.0243, 591.0747) -> (10.0479, 610.4794)
  line L109 (9.8386, 605.1872) -> (22.815, 585.7526)
  line L110 (23.0243, 591.0747) -> (10.0479, 610.4794)
  line L111 (9.8386, 605.1872) -> (22.815, 585.7526)
  line L112 (51.4287, 585.7526) -> (54.3887, 585.7526)
  line L113 (54.3887, 585.7526) -> (61.5645, 606.4729)
  line L114 (64.7339, 610.4794) -> (60.3387, 610.4794)
  line L115 (60.3387, 610.4794) -> (54.4186, 593.2873)
  line L116 (54.4186, 593.2873) -> (54.299, 593.0182)
  line L117 (54.299, 593.0182) -> (53.6113, 590.8953)
  line L118 (53.6113, 590.8953) -> (53.103, 589.3106)
  line L119 (61.5645, 606.4729) -> (61.5645, 585.7526)
  line L120 (61.5645, 585.7526) -> (64.7339, 585.7526)
  line L121 (64.7339, 585.7526) -> (64.7339, 610.4794)
  line L122 (61.5645, 606.4729) -> (61.5645, 585.7526)
  line L123 (61.5645, 585.7526) -> (64.7339, 585.7526)
  line L124 (64.7339, 585.7526) -> (64.7339, 610.4794)
  line L125 (46.0767, 610.4794) -> (41.1433, 610.4794)
  line L126 (41.1433, 610.4794) -> (41.1433, 585.7526)
  line L127 (41.1433, 585.7526) -> (44.2827, 585.7526)
  line L128 (44.2827, 585.7526) -> (44.2827, 606.8018)
  line L129 (53.103, 589.3106) -> (52.6246, 590.8056)
  line L130 (52.6246, 590.8056) -> (51.907, 592.9883)
  line L131 (51.907, 592.9883) -> (46.0767, 610.4794)
  line L132 (44.2827, 606.8018) -> (51.4287, 585.7526)
  line L133 (53.103, 589.3106) -> (52.6246, 590.8056)
  line L134 (52.6246, 590.8056) -> (51.907, 592.9883)
  line L135 (51.907, 592.9883) -> (46.0767, 610.4794)
  line L136 (44.2827, 606.8018) -> (51.4287, 585.7526)
  line L137 (87.9358, 610.4794) -> (70.056, 610.4794)
  line L138 (70.056, 610.4794) -> (70.056, 585.7526)
  line L139 (70.056, 585.7526) -> (88.5039, 585.7526)
  line L140 (88.5039, 585.7526) -> (88.5039, 588.6827)
  line L141 (88.5039, 588.6827) -> (73.3449, 588.6827)
  line L142 (73.3449, 588.6827) -> (73.3449, 597.1144)
  line L143 (73.3449, 597.1144) -> (87.0089, 597.1144)
  line L144 (87.0089, 597.1144) -> (87.0089, 600.0146)
  line L145 (87.0089, 600.0146) -> (73.3449, 600.0146)
  line L146 (73.3449, 600.0146) -> (73.3449, 607.5792)
  line L147 (73.3449, 607.5792) -> (87.9358, 607.5792)
  line L148 (87.9358, 607.5792) -> (87.9358, 610.4794)
  line L149 (110.1809, 610.4794) -> (92.4805, 610.4794)
  line L150 (92.4805, 610.4794) -> (92.4805, 607.5792)
  line L151 (92.4805, 607.5792) -> (106.2641, 607.5792)
  line L152 (106.2641, 607.5792) -> (105.0382, 606.2337)
  line L153 (105.0382, 606.2337) -> (103.7227, 604.649)
  line L154 (103.7227, 604.649) -> (91.0453, 588.8023)
  line L155 (91.0453, 588.8023) -> (91.0453, 585.7526)
  line L156 (91.0453, 585.7526) -> (110.5995, 585.7526)
  line L157 (110.5995, 585.7526) -> (110.5995, 588.6827)
  line L158 (110.5995, 588.6827) -> (94.8126, 588.6827)
  line L159 (94.8126, 588.6827) -> (96.3076, 590.4169)
  line L160 (96.3076, 590.4169) -> (110.1809, 607.5792)
  line L161 (110.1809, 607.5792) -> (110.1809, 610.4794)
  line L162 (118.5229, 595.9184) -> (121.2437, 603.1839)
  line L163 (121.2437, 603.1839) -> (121.5726, 604.0809)
  line L164 (121.5726, 604.0809) -> (122.1407, 605.9945)
  line L165 (122.1407, 605.9945) -> (122.5593, 607.908)
  line L166 (124.413, 610.4794) -> (120.8849, 610.4794)
  line L167 (120.8849, 610.4794) -> (111.4068, 585.7526)
  line L168 (111.4068, 585.7526) -> (114.8751, 585.7526)
  line L169 (114.8751, 585.7526) -> (117.5661, 593.2574)
  line L170 (117.5661, 593.2574) -> (127.9113, 593.2574)
  line L171 (127.9113, 593.2574) -> (130.7816, 585.7526)
  line L172 (130.7816, 585.7526) -> (134.519, 585.7526)
  line L173 (134.519, 585.7526) -> (124.413, 610.4794)
  line L174 (122.5593, 607.908) -> (122.9181, 606.7121)
  line L175 (122.9181, 606.7121) -> (123.5459, 604.8882)
  line L176 (123.5459, 604.8882) -> (124.3233, 602.7654)
  line L177 (124.3233, 602.7654) -> (126.8947, 595.9184)
  line L178 (126.8947, 595.9184) -> (118.5229, 595.9184)
  line L179 (-92.5368, 554.2985) -> (-89.816, 561.5341)
  line L180 (-89.816, 561.5341) -> (-89.4871, 562.461)
  line L181 (-89.4871, 562.461) -> (-88.919, 564.3447)
  line L182 (-88.919, 564.3447) -> (-88.4705, 566.2582)
  line L183 (-86.6466, 568.8595) -> (-90.1748, 568.8595)
  line L184 (-90.1748, 568.8595) -> (-99.6529, 544.1327)
  line L185 (-99.6529, 544.1327) -> (-96.1845, 544.1327)
  line L186 (-96.1845, 544.1327) -> (-93.4637, 551.6075)
  line L187 (-93.4637, 551.6075) -> (-83.1484, 551.6075)
  line L188 (-83.1484, 551.6075) -> (-80.2482, 544.1327)
  line L189 (-80.2482, 544.1327) -> (-76.5407, 544.1327)
  line L190 (-76.5407, 544.1327) -> (-86.6466, 568.8595)
  line L191 (-88.4705, 566.2582) -> (-88.1117, 565.0921)
  line L192 (-88.1117, 565.0921) -> (-87.5137, 563.2683)
  line L193 (-87.5137, 563.2683) -> (-86.7363, 561.1454)
  line L194 (-86.7363, 561.1454) -> (-84.1351, 554.2985)
  line L195 (-84.1351, 554.2985) -> (-92.5368, 554.2985)
  line L196 (-57.8237, 544.1327) -> (-54.4749, 544.1327)
  line L197 (-54.4749, 544.1327) -> (-54.4749, 568.8595)
  line L198 (-54.4749, 568.8595) -> (-57.6144, 568.8595)
  line L199 (-57.6144, 568.8595) -> (-57.6144, 549.4548)
  line L200 (-70.5907, 568.8595) -> (-73.9394, 568.8595)
  line L201 (-73.9394, 568.8595) -> (-73.9394, 544.1327)
  line L202 (-73.9394, 544.1327) -> (-70.8, 544.1327)
  line L203 (-70.8, 544.1327) -> (-70.8, 563.5673)
  line L204 (-57.6144, 549.4548) -> (-70.5907, 568.8595)
  line L205 (-70.8, 563.5673) -> (-57.8237, 544.1327)
  line L206 (-57.6144, 549.4548) -> (-70.5907, 568.8595)
  line L207 (-70.8, 563.5673) -> (-57.8237, 544.1327)
  line L208 (-32.2298, 546.5246) -> (-30.9142, 548.0495)
  line L209 (-30.9142, 548.0495) -> (-30.8843, 548.0794)
  line L210 (-30.8843, 548.0794) -> (-29.9574, 549.6641)
  line L211 (-29.9574, 549.6641) -> (-29.21, 551.6374)
  line L212 (-29.21, 551.6374) -> (-28.9708, 552.6241)
  line L213 (-28.9708, 552.6241) -> (-28.6718, 554.5377)
  line L214 (-28.6718, 554.5377) -> (-28.5522, 556.6306)
  line L215 (-28.5522, 556.6306) -> (-28.5522, 556.7502)
  line L216 (-28.5522, 556.7502) -> (-28.6718, 558.8133)
  line L217 (-28.6718, 558.8133) -> (-29.0007, 560.7567)
  line L218 (-29.0007, 560.7567) -> (-29.5089, 562.5208)
  line L219 (-29.5089, 562.5208) -> (-30.077, 563.7168)
  line L220 (-30.077, 563.7168) -> (-31.1235, 565.3612)
  line L221 (-31.1235, 565.3612) -> (-32.4391, 566.7366)
  line L222 (-40.5119, 565.9293) -> (-40.0634, 565.9293)
  line L223 (-40.0634, 565.9293) -> (-37.8509, 565.7798)
  line L224 (-37.8509, 565.7798) -> (-36.2961, 565.421)
  line L225 (-36.2961, 565.421) -> (-35.9971, 565.3014)
  line L226 (-35.9971, 565.3014) -> (-34.4722, 564.255)
  line L227 (-34.4722, 564.255) -> (-33.1866, 562.6404)
  line L228 (-33.1866, 562.6404) -> (-33.067, 562.4311)
  line L229 (-33.067, 562.4311) -> (-32.4391, 560.8763)
  line L230 (-32.4391, 560.8763) -> (-32.0504, 558.9628)
  line L231 (-32.0504, 558.9628) -> (-31.9308, 556.6904)
  line L232 (-31.9308, 556.6904) -> (-31.9607, 555.6738)
  line L233 (-31.9607, 555.6738) -> (-32.1401, 553.6706)
  line L234 (-32.1401, 553.6706) -> (-32.5587, 551.9364)
  line L235 (-32.5587, 551.9364) -> (-33.3062, 550.2621)
  line L236 (-33.3062, 550.2621) -> (-34.3825, 548.797)
  line L237 (-34.3825, 548.797) -> (-34.831, 548.4083)
  line L238 (-34.831, 548.4083) -> (-36.5951, 547.5113)
  line L239 (-36.5951, 547.5113) -> (-38.2396, 547.1525)
  line L240 (-38.2396, 547.1525) -> (-40.4521, 547.0628)
  line L241 (-40.4521, 547.0628) -> (-45.7144, 547.0628)
  line L242 (-32.2298, 546.5246) -> (-30.9142, 548.0495)
  line L243 (-30.9142, 548.0495) -> (-30.8843, 548.0794)
  line L244 (-30.8843, 548.0794) -> (-29.9574, 549.6641)
  line L245 (-29.9574, 549.6641) -> (-29.21, 551.6374)
  line L246 (-29.21, 551.6374) -> (-28.9708, 552.6241)
  line L247 (-28.9708, 552.6241) -> (-28.6718, 554.5377)
  line L248 (-28.6718, 554.5377) -> (-28.5522, 556.6306)
  line L249 (-28.5522, 556.6306) -> (-28.5522, 556.7502)
  line L250 (-28.5522, 556.7502) -> (-28.6718, 558.8133)
  line L251 (-28.6718, 558.8133) -> (-29.0007, 560.7567)
  line L252 (-29.0007, 560.7567) -> (-29.5089, 562.5208)
  line L253 (-29.5089, 562.5208) -> (-30.077, 563.7168)
  line L254 (-30.077, 563.7168) -> (-31.1235, 565.3612)
  line L255 (-31.1235, 565.3612) -> (-32.4391, 566.7366)
  line L256 (-40.5119, 565.9293) -> (-40.0634, 565.9293)
  line L257 (-40.0634, 565.9293) -> (-37.8509, 565.7798)
  line L258 (-37.8509, 565.7798) -> (-36.2961, 565.421)
  line L259 (-36.2961, 565.421) -> (-35.9971, 565.3014)
  line L260 (-35.9971, 565.3014) -> (-34.4722, 564.255)
  line L261 (-34.4722, 564.255) -> (-33.1866, 562.6404)
  line L262 (-33.1866, 562.6404) -> (-33.067, 562.4311)
  line L263 (-33.067, 562.4311) -> (-32.4391, 560.8763)
  line L264 (-32.4391, 560.8763) -> (-32.0504, 558.9628)
  line L265 (-32.0504, 558.9628) -> (-31.9308, 556.6904)
  line L266 (-31.9308, 556.6904) -> (-31.9607, 555.6738)
  line L267 (-31.9607, 555.6738) -> (-32.1401, 553.6706)
  line L268 (-32.1401, 553.6706) -> (-32.5587, 551.9364)
  line L269 (-32.5587, 551.9364) -> (-33.3062, 550.2621)
  line L270 (-33.3062, 550.2621) -> (-34.3825, 548.797)
  line L271 (-34.3825, 548.797) -> (-34.831, 548.4083)
  line L272 (-34.831, 548.4083) -> (-36.5951, 547.5113)
  line L273 (-36.5951, 547.5113) -> (-38.2396, 547.1525)
  line L274 (-38.2396, 547.1525) -> (-40.4521, 547.0628)
  line L275 (-40.4521, 547.0628) -> (-45.7144, 547.0628)
  line L276 (-32.4391, 566.7366) -> (-32.5587, 566.8263)
  line L277 (-32.5587, 566.8263) -> (-34.1732, 567.8429)
  line L278 (-34.1732, 567.8429) -> (-36.0868, 568.5007)
  line L279 (-36.0868, 568.5007) -> (-36.4157, 568.5904)
  line L280 (-36.4157, 568.5904) -> (-38.1798, 568.7997)
  line L281 (-38.1798, 568.7997) -> (-40.482, 568.8595)
  line L282 (-45.7144, 547.0628) -> (-45.7144, 565.9293)
  line L283 (-45.7144, 565.9293) -> (-40.5119, 565.9293)
  line L284 (-40.482, 568.8595) -> (-48.9734, 568.8595)
  line L285 (-48.9734, 568.8595) -> (-48.9734, 544.1327)
  line L286 (-48.9734, 544.1327) -> (-40.0634, 544.1327)
  line L287 (-40.0634, 544.1327) -> (-40.0036, 544.1327)
  line L288 (-40.0036, 544.1327) -> (-37.9107, 544.2523)
  line L289 (-37.9107, 544.2523) -> (-36.0868, 544.5513)
  line L290 (-36.0868, 544.5513) -> (-34.831, 544.94)
  line L291 (-34.831, 544.94) -> (-33.1567, 545.807)
  line L292 (-33.1567, 545.807) -> (-32.2298, 546.5246)
  line L293 (-16.9512, 555.1058) -> (-15.1273, 554.9862)
  line L294 (-15.1273, 554.9862) -> (-13.6324, 554.3284)
  line L295 (-13.6324, 554.3284) -> (-13.3932, 554.1789)
  line L296 (-13.3932, 554.1789) -> (-11.9879, 552.6839)
  line L297 (-11.9879, 552.6839) -> (-11.8982, 552.5643)
  line L298 (-11.8982, 552.5643) -> (-10.8517, 551.159)
  line L299 (-10.8517, 551.159) -> (-9.6259, 549.2754)
  line L300 (-9.6259, 549.2754) -> (-6.3369, 544.1327)
  line L301 (-6.3369, 544.1327) -> (-2.2407, 544.1327)
  line L302 (-2.2407, 544.1327) -> (-6.5163, 550.86)
  line L303 (-6.5163, 550.86) -> (-6.7256, 551.159)
  line L304 (-6.7256, 551.159) -> (-7.9515, 552.8035)
  line L305 (-7.9515, 552.8035) -> (-9.2372, 554.149)
  line L306 (-9.2372, 554.149) -> (-9.4764, 554.3284)
  line L307 (-9.4764, 554.3284) -> (-11.2105, 555.3748)
  line L308 (-16.9512, 555.1058) -> (-15.1273, 554.9862)
  line L309 (-15.1273, 554.9862) -> (-13.6324, 554.3284)
  line L310 (-13.6324, 554.3284) -> (-13.3932, 554.1789)
  line L311 (-13.3932, 554.1789) -> (-11.9879, 552.6839)
  line L312 (-11.9879, 552.6839) -> (-11.8982, 552.5643)
  line L313 (-11.8982, 552.5643) -> (-10.8517, 551.159)
  line L314 (-10.8517, 551.159) -> (-9.6259, 549.2754)
  line L315 (-9.6259, 549.2754) -> (-6.3369, 544.1327)
  line L316 (-6.3369, 544.1327) -> (-2.2407, 544.1327)
  line L317 (-2.2407, 544.1327) -> (-6.5163, 550.86)
  line L318 (-6.5163, 550.86) -> (-6.7256, 551.159)
  line L319 (-6.7256, 551.159) -> (-7.9515, 552.8035)
  line L320 (-7.9515, 552.8035) -> (-9.2372, 554.149)
  line L321 (-9.2372, 554.149) -> (-9.4764, 554.3284)
  line L322 (-9.4764, 554.3284) -> (-11.2105, 555.3748)
  line L323 (-5.9482, 557.6771) -> (-5.3204, 558.4545)
  line L324 (-5.3204, 558.4545) -> (-4.5131, 560.1587)
  line L325 (-4.5131, 560.1587) -> (-4.244, 562.1022)
  line L326 (-4.244, 562.1022) -> (-4.244, 562.1321)
  line L327 (-4.244, 562.1321) -> (-4.5131, 564.0756)
  line L328 (-4.5131, 564.0756) -> (-5.2905, 565.8396)
  line L329 (-5.2905, 565.8396) -> (-6.4266, 567.215)
  line L330 (-12.9148, 566.1386) -> (-12.4065, 566.1087)
  line L331 (-12.4065, 566.1087) -> (-10.3434, 565.7798)
  line L332 (-10.3434, 565.7798) -> (-8.8784, 565.0024)
  line L333 (-8.8784, 565.0024) -> (-8.0711, 563.956)
  line L334 (-8.0711, 563.956) -> (-7.6226, 562.1022)
  line L335 (-7.6226, 562.1022) -> (-7.6525, 561.7135)
  line L336 (-7.6525, 561.7135) -> (-8.2804, 559.8897)
  line L337 (-8.2804, 559.8897) -> (-8.6093, 559.4711)
  line L338 (-8.6093, 559.4711) -> (-10.1939, 558.4246)
  line L339 (-10.1939, 558.4246) -> (-11.5394, 558.0957)
  line L340 (-11.5394, 558.0957) -> (-13.7221, 557.9462)
  line L341 (-13.7221, 557.9462) -> (-20.7484, 557.9462)
  line L342 (-6.4266, 567.215) -> (-8.0412, 568.2017)
  line L343 (-8.0412, 568.2017) -> (-8.9083, 568.4708)
  line L344 (-8.9083, 568.4708) -> (-10.7321, 568.7698)
  line L345 (-10.7321, 568.7698) -> (-13.0643, 568.8595)
  line L346 (-20.7484, 557.9462) -> (-20.7484, 566.1386)
  line L347 (-20.7484, 566.1386) -> (-12.9148, 566.1386)
  line L348 (-11.2105, 555.3748) -> (-11.1806, 555.3748)
  line L349 (-11.1806, 555.3748) -> (-9.0279, 555.8532)
  line L350 (-9.0279, 555.8532) -> (-7.2937, 556.6306)
  line L351 (-7.2937, 556.6306) -> (-5.9482, 557.6771)
  line L352 (-13.0643, 568.8595) -> (-24.0075, 568.8595)
  line L353 (-24.0075, 568.8595) -> (-24.0075, 544.1327)
  line L354 (-24.0075, 544.1327) -> (-20.7484, 544.1327)
  line L355 (-20.7484, 544.1327) -> (-20.7484, 555.1058)
  line L356 (-20.7484, 555.1058) -> (-16.9512, 555.1058)
  line L357 (18.8084, 568.8595) -> (0.9286, 568.8595)
  line L358 (0.9286, 568.8595) -> (0.9286, 544.1327)
  line L359 (0.9286, 544.1327) -> (19.3765, 544.1327)
  line L360 (19.3765, 544.1327) -> (19.3765, 547.0628)
  line L361 (19.3765, 547.0628) -> (4.2175, 547.0628)
  line L362 (4.2175, 547.0628) -> (4.2175, 555.4645)
  line L363 (4.2175, 555.4645) -> (17.8816, 555.4645)
  line L364 (17.8816, 555.4645) -> (17.8816, 558.3648)
  line L365 (17.8816, 558.3648) -> (4.2175, 558.3648)
  line L366 (4.2175, 558.3648) -> (4.2175, 565.9293)
  line L367 (4.2175, 565.9293) -> (18.8084, 565.9293)
  line L368 (18.8084, 565.9293) -> (18.8084, 568.8595)
  line L369 (33.1601, 546.6442) -> (31.1868, 546.8236)
  line L370 (31.1868, 546.8236) -> (29.3629, 547.3917)
  line L371 (29.3629, 547.3917) -> (28.1968, 548.0196)
  line L372 (28.1968, 548.0196) -> (26.8813, 549.3053)
  line L373 (26.8813, 549.3053) -> (26.3431, 550.3518)
  line L374 (26.3431, 550.3518) -> (25.8647, 552.355)
  line L375 (25.8647, 552.355) -> (22.7851, 552.0859)
  line L376 (22.7851, 552.0859) -> (22.8449, 551.2487)
  line L377 (22.8449, 551.2487) -> (23.2933, 549.3651)
  line L378 (23.2933, 549.3651) -> (24.1305, 547.6309)
  line L379 (24.1305, 547.6309) -> (24.6089, 547.003)
  line L380 (24.6089, 547.003) -> (25.9843, 545.6576)
  line L381 (25.9843, 545.6576) -> (27.6886, 544.7008)
  line L382 (27.6886, 544.7008) -> (29.2433, 544.1626)
  line L383 (29.2433, 544.1626) -> (31.1569, 543.8337)
  line L384 (31.1569, 543.8337) -> (33.3096, 543.7141)
  line L385 (33.3096, 543.7141) -> (34.3561, 543.744)
  line L386 (34.3561, 543.744) -> (36.2996, 544.0729)
  line L387 (36.2996, 544.0729) -> (38.0935, 544.7008)
  line L388 (38.0935, 544.7008) -> (38.4523, 544.8802)
  line L389 (38.4523, 544.8802) -> (40.0968, 545.9864)
  line L390 (40.0968, 545.9864) -> (41.3227, 547.3917)
  line L391 (41.3227, 547.3917) -> (41.3526, 547.4515)
  line L392 (41.3526, 547.4515) -> (42.1599, 549.2156)
  line L393 (42.1599, 549.2156) -> (42.4588, 551.1291)
  line L394 (42.4588, 551.1291) -> (42.2197, 552.9231)
  line L395 (42.2197, 552.9231) -> (41.4124, 554.6274)
  line L396 (41.4124, 554.6274) -> (41.3227, 554.7769)
  line L397 (41.3227, 554.7769) -> (40.037, 556.0924)
  line L398 (40.037, 556.0924) -> (38.243, 557.1389)
  line L399 (38.243, 557.1389) -> (37.077, 557.5874)
  line L400 (37.077, 557.5874) -> (35.2232, 558.1256)
  line L401 (35.2232, 558.1256) -> (32.7715, 558.7535)
  line L402 (32.7715, 558.7535) -> (30.9177, 559.202)
  line L403 (30.9177, 559.202) -> (28.9443, 559.8598)
  line L404 (28.9443, 559.8598) -> (27.8381, 560.4876)
  line L405 (27.8381, 560.4876) -> (27.4494, 560.9062)
  line L406 (27.4494, 560.9062) -> (26.8813, 562.7002)
  line L407 (26.8813, 562.7002) -> (27.0607, 563.7766)